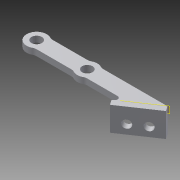
# Autodesk Inventor part: leg
Saved by Autodesk Inventor 2014 (Build 180170000, 170)
## iProperties
Created: 2015-03-09
Part Number: leg
Material: 一般
Document SubType Name: Modeling
Designer: Hideyuki Takei
Density: 1 g/cm^3
Appearance: 既定
d0: 4.000 mm
d1: 45.000 mm
d2: 5.200 mm
d3: 5.200 mm
d4: 25.100 mm
d5: 3.000 mm
d6: 0.00 deg
d7: 12.163 mm
d8: 8.000 mm
d9: 4.000 mm
d10: 56.00 deg
d11: 0.000 mm
d12: 20.000 mm
d13: 0.000 mm
d14: 12.000 mm
d15: 1.500 mm
d19: 4.000 mm
d21: 4.000 mm
d22: 4.000 mm
d23: 5.600 mm
d24: 6.000 mm
d25: 6.000 mm
d26: 6.000 mm
d28: 6.000 mm
d29: 6.000 mm
d30: 6.000 mm
d31: 3.000 mm
d32: 0.00 deg
d34: 10.000 mm
d35: 10.000 mm
d36: 3.000 mm
d39: 0.000 mm
d40: 1.500 mm
Author: Hideyuki Takei
Autodesk Inventor part; units mm, degrees
note: some values were not read from the file. Chosen so that the rebuilt part matches the saved one: sketch regions of "押し出し1".
ref_plane "YZ Plane" through (0, 0, 0) normal (1, 0, 0) x (0, 1, 0)
ref_plane "XZ Plane" through (0, 0, 0) normal (0, 1, 0) x (-1, 0, 0)
ref_plane "XY Plane" through (0, 0, 0) normal (0, 0, 1) x (1, 0, 0)
sketch "スケッチ1" plane through (0, 0, 0) normal (0, 0, 1) x (1, 0, 0)
  line L0 (0, 0) -> (45, 0) construction
  line L1 (0, -4) -> (45, -4)
  line L2 (45, 4) -> (0, 4)
  arc A0 (0, 4) -> (0, -4) centre (0, 0) ccw
  arc A1 (45, -4) -> (45, 4) centre (45, 0) ccw
  circle A2 centre (0, 0) radius 2.6
  circle A3 centre (25.1, 0) radius 2.6
  line L3 (36.8368, 4) -> (49, 4)
  line L4 (49, 4) -> (49, -4)
  line L5 (49, -4) -> (36.8368, -4)
  line L6 (36.8368, -4) -> (36.8368, 4)
  circle A4 centre (0, 0) radius 5
  circle A5 centre (25.1, 0) radius 5
  point P0 (22.5, 0)
  dimension "d0" = 4
  dimension "d1" = 45
  dimension "d2" = 5.2
  dimension "d3" = 5.2
  dimension "d4" = 25.1
  dimension "d7" = 12.1632
  dimension "d8" = 8
  dimension "d9" = 4
  dimension "d34" = 10
  dimension "d35" = 10
  constraints: 16 end point, 6 centre point, 4 point on circle, 4 tangent, 3 coincident, 3 parallel, 2 horizontal, 2 point on line, 1 midpoint, 1 perpendicular
  measures "d0" radius of A0
  measures "d1" distance of L0.start L0.end
  measures "d2" diameter of A2
  measures "d3" diameter of A3
  measures "d4" distance of L0.start A3.centre
  measures "d7" distance of L4.end L5.end
  measures "d8" distance of L3.end L4.end
  measures "d9" distance from line of L4 L0.end
  measures "d34" diameter of A4
  measures "d35" diameter of A5
extrude "押し出し1" add sketch "スケッチ1" along normal blind 3
draft "面の勾配1" angle 56 pull direction (0, -1, 0) faces at (49, -1.3333, 1) fixed edges at (49, -4, 1.5)
ref_plane "作業平面1" through (60.8605, 4, 0) normal (0.5591929, -0.8290376, 0) x (0.8290376, 0.5591929, 0)
sketch "スケッチ3" plane through (60.8605, 4, 0) normal (0.5591929, -0.8290376, 0) x (0.8290376, 0.5591929, 0)
  line L0 (0, -9) -> (-20, -9)
  line L1 (-20, -9) -> (-20, 3)
  line L2 (-20, 3) -> (0, 3)
  line L3 (0, 3) -> (0, -9)
  line L4 (0, 0) -> (0, 3) projected
  circle A0 centre (-14, -4.5) radius 2
  circle A1 centre (-6, -4.5) radius 2
  line L5 (-31.6332, 3) -> (-14.3063, 3) projected
  point P0 (-52.6924, 0)
  point P1 (2.1488, 1.5)
  dimension "d12" = 20
  dimension "d13" = 0
  dimension "d14" = 12
  dimension "d15" = 1.5
  dimension "d21" = 4
  dimension "d22" = 4
  dimension "d25" = 6
  dimension "d26" = 6
  dimension "d29" = 6
  dimension "d30" = 6
  dimension "d39" = 0
  constraints: 8 end point, 2 centre point, 2 parallel, 1 horizontal, 1 perpendicular
  measures "d12" distance of L1.end L2.end
  measures "d13" distance between parallel lines of L4 L3
  measures "d14" distance of L2.end L0.start
  measures "d15" vertical distance of point (2.149, 1.5) L4.start
  measures "d21" diameter of A0
  measures "d22" diameter of A1
  measures "d25" vertical distance of point (2.149, 1.5) A0.centre
  measures "d26" vertical distance of point (2.149, 1.5) A1.centre
  measures "d29" distance from line of A1.centre L3
  measures "d30" distance from line of L1 A0.centre
  measures "d39" distance between parallel lines of L2 L5
extrude "押し出し3" add sketch "スケッチ3" along normal blind 3
fillet "フィレット2" radius 3 6 edges at (3, 4, 1.5) (28.1, 4, 1.5) (22.1, 4, 1.5) (3, -4, 1.5) (28.1, -4, 1.5) (22.1, -4, 1.5)
fillet "フィレット5" radius 1.5 2 edges at (54.9302, 0, 0) (49, -4, 1.5)
equation "\"d3\" = d2"
equation "\"d21\" = d19"
equation "\"d22\" = d19"
equation "\"d26\" = d25"
equation "\"d29\" = d28"
equation "\"d30\" = d24"
equation "\"d28\" = d24"
equation "\"d19\" = 4"
equation "\"d24\" = 6"
